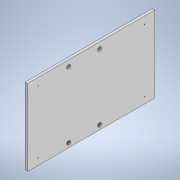
# Autodesk Inventor part: exp base 1
Saved by Autodesk Inventor 2020 (Build 240168000, 168)
## iProperties
Created: 2020-02-18
Part Number: exp base 1
Material: Generic
Document SubType Name: Modeling
Designer: Hp
Density: 1 g/cm^3
Appearance: Default
Author: Hp
Autodesk Inventor part; units mm, degrees
ref_plane "YZ Plane" through (0, 0, 0) normal (1, 0, 0) x (0, 1, 0)
ref_plane "XZ Plane" through (0, 0, 0) normal (0, 1, 0) x (-1, 0, 0)
ref_plane "XY Plane" through (0, 0, 0) normal (0, 0, 1) x (1, 0, 0)
sketch "Sketch1" plane through (0, 0, 0) normal (1, 0, 0) x (0, 1, 0)
  line L0 (4.324, 13.8845) -> (-295.676, 13.8845)
  line L1 (-295.676, 13.8845) -> (-295.676, -486.1155)
  line L2 (-295.676, -486.1155) -> (4.324, -486.1155)
  line L3 (4.324, -486.1155) -> (4.324, 13.8845)
  point P0 (0, 0)
  dimension "d0" = 300
  dimension "d1" = 500
  constraints: 8 end point, 2 parallel, 1 horizontal, 1 perpendicular
  measures "d0" distance of L2.end L1.end
  measures "d1" distance of L1.end L0.end
extrude "Extrusion1" add sketch "Sketch1" along normal blind 10
sketch "Sketch2" plane through (10, 0, 0) normal (1, 0, 0) x (0, 0, -1)
  line L0 (27.0974, -24.4856) -> (445.6374, -24.4856)
  line L1 (445.6374, -24.4856) -> (445.6374, -270.6472)
  line L2 (445.6374, -270.6472) -> (27.0974, -270.6472)
  line L3 (27.0974, -270.6472) -> (27.0974, -24.4856)
  point P0 (0, 0)
  constraints: 8 end point, 2 parallel, 1 horizontal, 1 perpendicular
hole "Hole1" at (10, -24.4856, -27.0974) at (10, -24.4856, -445.6374) at (10, -270.6472, -445.6374) at (10, -270.6472, -27.0974) direction (-1, 0, 0) diameter 3 end through all
sketch "Sketch4" plane through (10, 0, 0) normal (1, 0, 0) x (0, 0, -1)
  point P0 (0, 0)
sketch "Sketch9" plane through (10, 0, 0) normal (1, 0, 0) x (0, 0, -1)
  circle A0 centre (146.7684, -19.2122) radius 7.5 projected
  line L0 (146.7684, -19.2122) -> (268.3405, -19.2122)
  line L1 (268.3405, -19.2122) -> (268.3405, -278.104)
  line L2 (268.3405, -278.104) -> (146.7684, -278.104)
  line L3 (146.7684, -278.104) -> (146.7684, -19.2122)
  point P0 (0, 0)
  constraints: 8 end point, 2 parallel, 1 horizontal, 1 perpendicular
hole "Hole7" at (10, -19.2122, -146.7684) at (10, -19.2122, -268.3405) at (10, -278.104, -146.7684) at (10, -278.104, -268.3405) direction (-1, 0, 0) diameter 15 end through all
body "Solid1"
